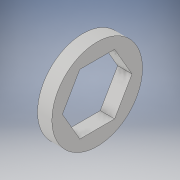
# Autodesk Inventor part: 3D Model Spacer
Saved by Autodesk Inventor 2018 (Build 220112000, 112)
## iProperties
Created: 2019-01-23
Part Number: 3D Model Spacer
Material: Generic
Document SubType Name: Modeling
Designer: Gabriel
Density: 1 g/cm^3
Appearance: Default
Author: Gabriel
Autodesk Inventor part; units mm, degrees
ref_plane "YZ Plane" through (0, 0, 0) normal (1, 0, 0) x (0, 1, 0)
ref_plane "XZ Plane" through (0, 0, 0) normal (0, 1, 0) x (-1, 0, 0)
ref_plane "XY Plane" through (0, 0, 0) normal (0, 0, 1) x (1, 0, 0)
sketch "Sketch1" plane through (0, 0, 0) normal (1, 0, 0) x (0, 1, 0)
  circle A0 centre (5.9226, 5.0314) radius 9.525
  line L0 (5.9226, 5.0314) -> (12.2726, 5.0314) construction
  line L1 (12.2726, 1.3724) -> (5.9287, -2.2974)
  line L2 (5.9287, -2.2974) -> (-0.4213, 1.3617)
  line L3 (-0.4213, 1.3617) -> (-0.4274, 8.6905)
  line L4 (-0.4274, 8.6905) -> (5.9164, 12.3602)
  line L5 (5.9164, 12.3602) -> (12.2664, 8.7012)
  line L6 (12.2664, 8.7012) -> (12.2726, 1.3724)
  point P0 (0, 0)
  dimension "d0" = 19.05
  constraints: 14 end point, 1 centre point, 1 coincident, 1 horizontal, 13 other
  measures "d0" diameter of A0
extrude "Extrusion1" add sketch "Sketch1" along normal blind 3.0226
body "Solid1"
